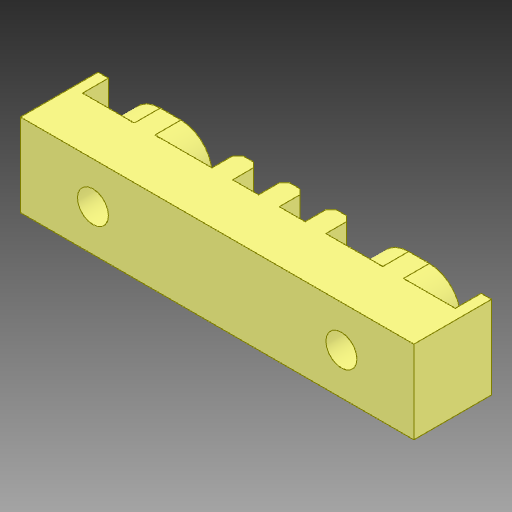
# Autodesk Inventor part: Dribblerdaempfer
Saved by Autodesk Inventor 2019.4 (Build 234330000, 330)
## iProperties
Part Number: Dribblerdaempfer
Material: Gummi, Silikon
Document SubType Name: Modeling
Designer: rYan
Density: 1.25 g/cm^3
Appearance: Gummi - Schwarz
Mass: 2.04661 g
Surface Area: 16.3403 cm^2
Volume: 1.63729 cm^3
Author: rYan
Autodesk Inventor part; units mm, degrees
ref_plane "YZ Plane" through (0, 0, 0) normal (1, 0, 0) x (0, 1, 0)
ref_plane "XZ Plane" through (0, 0, 0) normal (0, 1, 0) x (-1, 0, 0)
ref_plane "XY Plane" through (0, 0, 0) normal (0, 0, 1) x (1, 0, 0)
sketch "Skizze1" plane through (0, 0, 0) normal (0, 0, 1) x (1, 0, 0)
  line L0 (-19, 0) -> (19, 0)
  line L1 (19, 0) -> (19, 7.5)
  line L2 (-19, 7.5) -> (-19, 0)
  line L3 (0, 9) -> (0, -1.5) projected
  line L4 (19, 7.5) -> (18, 7.5)
  line L5 (18, 7.5) -> (18, 5)
  line L6 (-18, 5) -> (-18, 7.5)
  line L7 (-18, 7.5) -> (-19, 7.5)
  line L8 (-12, 7.5) -> (-12, 0) construction
  line L9 (12, 7.5) -> (12, 0) construction
  line L10 (-16, 5) -> (-16, 7.5)
  line L11 (-16, 7.5) -> (-8, 7.5)
  line L12 (-8, 7.5) -> (-8, 5)
  line L13 (16, 5) -> (16, 7.5)
  line L14 (16, 7.5) -> (8, 7.5)
  line L15 (8, 7.5) -> (8, 5)
  line L16 (-16, 5) -> (-18, 5)
  line L17 (18, 5) -> (16, 5)
  line L18 (8, 5) -> (-8, 5)
  point P0 (0, 0)
  dimension "d0" = 38
  dimension "d1" = 7.5
  dimension "d34" = 2.5
  dimension "d35" = 24
  dimension "d36" = 8
  dimension "d37" = 1
  constraints: 36 end point, 16 perpendicular, 5 horizontal, 4 point on line, 3 collinear, 3 midpoint, 3 parallel, 1 vertical, 7 other
  measures "d0" distance of L0.start L0.end
  measures "d1" distance of L0.end L1.end
  measures "d34" distance of L4.end L5.end
  measures "d35" distance between parallel lines of L9 L8
  measures "d36" distance of L13.end L14.end
  measures "d37" distance of L1.end L4.end
extrude "Extrusion1" add sketch "Skizze1" along normal blind 8
sketch "Skizze5" plane through (8, 7.5, 0) normal (0, 1, 0) x (1, 0, 0)
  line L0 (8, 0) -> (0, 0) projected
  line L1 (0, 0) -> (0, -8) projected
  line L2 (8, -8) -> (0, -8) projected
  line L3 (8, 0) -> (8, -8) projected
  line L4 (-16, 0) -> (-24, 0) projected
  line L5 (-24, 0) -> (-24, -8) projected
  line L6 (-16, -8) -> (-24, -8) projected
  line L7 (-16, 0) -> (-16, -8) projected
  line L8 (-27, -8) -> (11, -8) construction
  line L9 (4, -8) -> (4, 0) construction
  line L10 (-27, 0) -> (11, 0) construction
  line L11 (-20, 0) -> (-20, -8) construction
  point P0 (-8, 0)
  point P1 (4, -4)
  point P2 (-20, -4)
  constraints: 4 end point, 4 midpoint, 2 vertical, 1 point on line, 2 other
hole "Bohrung2" at (12, 7.5, 4) at (-12, 7.5, 4) direction (0, -1, 0) diameter 3 end through all counterbore diameter 6 counterbore depth 5
sketch "Skizze6" plane through (0, 0, 8) normal (0, 0, 1) x (1, 0, 0)
  line L0 (0, 9) -> (0, -1.5) projected
  line L1 (8, 5) -> (-8, 5) projected
  line L2 (8, 5) -> (-8, 5) projected
  line L3 (8, 5) -> (-8, 5) projected
  line L4 (-1, 5) -> (1, 5)
  line L5 (1, 5) -> (1, 7.5)
  line L6 (1, 7.5) -> (-1, 7.5)
  line L7 (-1, 7.5) -> (-1, 5)
  line L8 (16, 7.5) -> (8, 7.5) projected
  point P0 (0, 0)
  dimension "d45" = 2
  constraints: 8 end point, 2 parallel, 1 collinear, 1 horizontal, 1 perpendicular, 1 point on line, 1 other
  measures "d45" distance of L5.end L6.end
extrude "Extrusion4" add sketch "Skizze6" against normal up to surface (8 mm away)
pattern_linear "Rechteckige Anordnung2" count 3 spacing 4.5 along (-1, 0, 0) of "Extrusion4" first direction both ways yes
fillet "Rundung1" radius 3 8 edges at (8, 6.25, 8) (16, 6.25, 8) (16, 6.25, 0) (8, 6.25, 0) (-8, 6.25, 0) (-16, 6.25, 0) (-16, 6.25, 8) (-8, 6.25, 8)
chamfer "Fase1" distance 0.5 angle 45 6 edges at (3.5, 7.5, 4) (5.5, 7.5, 4) (1, 7.5, 4) (-1, 7.5, 4) (-3.5, 7.5, 4) (-5.5, 7.5, 4)
